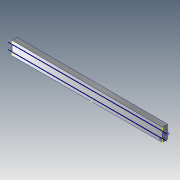
# Autodesk Inventor part: Y table support
Saved by Autodesk Inventor 2019 (Build 230136000, 136)
## iProperties
Created: 2018-10-20
Part Number: Y table support
Material: Aluminum 6061
Document SubType Name: Modeling
Designer: LillaHunden
Density: 2.7 g/cm^3
Appearance: Aluminum - Flat
Mass: 304.022 g
Surface Area: 289.886 cm^2
Volume: 112.601 cm^3
Author: LillaHunden
Autodesk Inventor part; units mm, degrees
ref_plane "YZ Plane" through (0, 0, 0) normal (1, 0, 0) x (0, 1, 0)
ref_plane "XZ Plane" through (0, 0, 0) normal (0, 1, 0) x (-1, 0, 0)
ref_plane "XY Plane" through (0, 0, 0) normal (0, 0, 1) x (1, 0, 0)
sketch "Sketch1" plane through (0, 0, 0) normal (0, 0, 1) x (1, 0, 0)
  line L0 (127.75, 2.5629) -> (108.85, 2.5629) construction
  line L1 (-186.25, 0) -> (133.75, 0) construction
  line L2 (133.75, 0) -> (133.75, 5) construction
  line L3 (-186.25, 5) -> (133.75, 5) construction
  line L4 (-186.25, 0) -> (-186.25, 5) construction
  line L5 (133.75, 0) -> (-186.25, 0)
  line L6 (-186.25, 0) -> (-186.25, 25)
  line L7 (-186.25, 25) -> (133.75, 25)
  line L8 (133.75, 25) -> (133.75, 0)
  line L9 (-186.25, 0) -> (-186.25, 5)
  dimension "d1" = 25
  constraints: 20 end point, 2 parallel, 1 horizontal, 1 perpendicular
  measures "d1" distance of L5.end L6.end
extrude "Extrusion1" add sketch "Sketch1" along normal blind 9.9823
sketch "Sketch2" plane through (-186.25, 0, 0) normal (-1, 0, 0) x (0, 0, 1)
  line L0 (0, 0) -> (0, 25) projected
  line L1 (0, 0) -> (9.9823, 0) projected
  line L2 (9.9823, 25) -> (9.9823, 0) projected
  line L3 (0, 25) -> (9.9823, 25) projected
  point P0 (0, 0)
extrude "Extrusion2" cut sketch "Sketch2" against normal blind 36
sketch "Sketch3" plane through (0, 0, 9.9823) normal (0, 0, 1) x (1, 0, 0)
  line L0 (-157.75, 6.5) -> (141.25, 6.5)
  line L1 (141.25, 18.5) -> (-157.75, 18.5)
  line L2 (-150.25, 25) -> (-150.25, 0) projected
  line L3 (133.75, 0) -> (133.75, 25) projected
  line L4 (-150.25, 19) -> (133.75, 19)
  line L5 (133.75, 19) -> (133.75, 6)
  line L6 (133.75, 6) -> (-150.25, 6)
  line L7 (-150.25, 6) -> (-150.25, 19)
  point P0 (0, 0)
  dimension "d6" = 0.5
  dimension "d7" = 0.5
  constraints: 12 end point, 3 horizontal, 2 parallel, 2 point on line, 1 perpendicular, 4 other
  measures "d6" distance between parallel lines of L1 L4
  measures "d7" distance between parallel lines of L6 L0
extrude "Extrusion3" cut sketch "Sketch3" against normal blind 2
body "Solid1"
